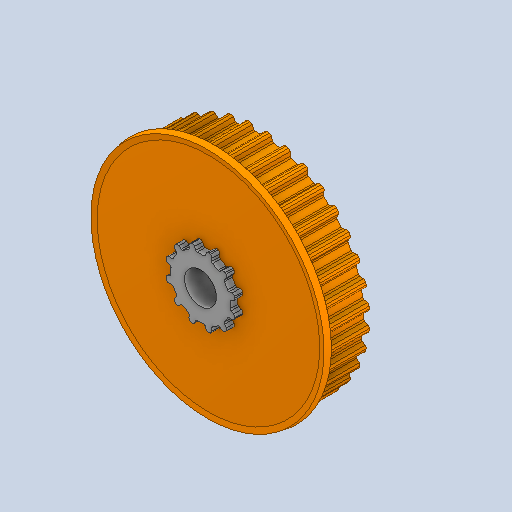
# Autodesk Inventor part: Synchronous Pulley2
Saved by Autodesk Inventor 2022.2 (Build 262287000, 287)
## iProperties
CustomPartVersion: 1
Created: 2022-01-04
Part Number: Synchronous Pulley2
Material: Steel
Document SubType Name: Modeling
Designer: Jochen
Density: 1 g/cm^3
Appearance: Steel
Author: Jochen
Autodesk Inventor part; units mm, degrees
ref_plane "YZ Plane" through (0, 0, 0) normal (1, 0, 0) x (0, 1, 0)
ref_plane "XZ Plane" through (0, 0, 0) normal (0, 1, 0) x (-1, 0, 0)
ref_plane "XY Plane" through (0, 0, 0) normal (0, 0, 1) x (1, 0, 0)
sketch "Pulley Sketch" plane through (0, 0, 0) normal (0, 0, 1) x (1, 0, 0)
  circle A0 centre (0, 0) radius 14.3239 construction
  circle A1 centre (0, 0) radius 14.0239
  circle A2 centre (0, 0) radius 13.2739
  line L0 (-0.8624, 13.9974) -> (-0.525, 13.2739)
  line L1 (-0.525, 13.2739) -> (0.525, 13.2739)
  line L2 (0.525, 13.2739) -> (0.8624, 13.9974)
  line L3 (0, 0) -> (0, 14.0239) construction
  point P0 (0, 13.2739)
  dimension "d0" = 28.6479
  dimension "d1" = 0.3
  dimension "d2" = 0.75
  dimension "d3" = 50
  dimension "d4" = 1.05
  constraints: 8 end point, 3 coincident, 3 point on circle, 2 centre point, 1 horizontal, 1 midpoint, 1 point on line, 1 vertical, 1 vertical alignment, 3 other
  measures "d0" diameter of A0
  measures "d1" radial gap between concentric circles of A0 A1
  measures "d3" angle of L2 L0
  measures "d4" distance of L0.end L1.end
extrude "Base Body" add sketch "Pulley Sketch" along normal mid plane 5.5 contours A2 | A1 L0 L1 L2 | L2 L1 L0 A1
extrude "Tooth" cut sketch "Pulley Sketch" along normal through all both and the other way through all contours L2 L1 L0 A1 picked at (0, 13.7719)
fillet "Tooth Fillet" radius 0.2 2 edges at (0.525, 13.2739, 0) (-0.525, 13.2739, 0)
fillet "Tooth Fillet" radius 0.3 4 edges at (-0.8624, 13.9974, 1.375) (-0.8624, 13.9974, -1.375) (0.8624, 13.9974, 1.375) (0.8624, 13.9974, -1.375)
pattern_circular "Teeth" count 36 over 360 about axis through (0, 0, -10) along (0, 0, 1) of "Tooth", "Tooth Fillet"
feature "Left flange" [suppressed]
pulley flange "Right flange" diameter 28.0479 height 0.8 thickness 0.8 bend angle 10 centre (0, 0, 2.75) toward (0, 0, 1)
sketch "Sketch2" plane through (0, 0, -2.75) normal (0, 0, -1) x (-1, 0, 0)
  circle A0 centre (0, 0) radius 17.5
  circle A1 centre (0, 0) radius 2
  arc A2 (-3.1617, 13.4663) -> (-3.482, 13.5848) centre (-3.4075, 13.2942) ccw projected
  arc A3 (-3.482, 13.5848) -> (-3.7769, 13.5058) centre (0, 0) ccw projected
  arc A4 (-3.7769, 13.5058) -> (-3.995, 13.243) centre (-3.6961, 13.2169) ccw projected
  line L0 (-3.995, 13.243) -> (-4.0355, 12.7799) projected
  arc A5 (-4.1663, 12.6094) -> (-4.0355, 12.7799) centre (-4.2348, 12.7973) ccw projected
  line L1 (-4.1663, 12.6094) -> (-4.9136, 12.3374) projected
  arc A6 (-5.1234, 12.384) -> (-4.9136, 12.3374) centre (-4.982, 12.5254) ccw projected
  line L2 (-5.1234, 12.384) -> (-5.4521, 12.7127) projected
  arc A7 (-5.4521, 12.7127) -> (-5.788, 12.7738) centre (-5.6642, 12.5005) ccw projected
  arc A8 (-5.788, 12.7738) -> (-6.0648, 12.6447) centre (0, 0) ccw projected
  arc A9 (-6.0648, 12.6447) -> (-6.2339, 12.3481) centre (-5.9351, 12.3742) ccw projected
  line L3 (-6.2339, 12.3481) -> (-6.1934, 11.885) projected
  arc A10 (-6.2927, 11.6944) -> (-6.1934, 11.885) centre (-6.3927, 11.8676) ccw projected
  line L4 (-6.2927, 11.6944) -> (-6.9813, 11.2968) projected
  arc A11 (-7.196, 11.3062) -> (-6.9813, 11.2968) centre (-7.0813, 11.47) ccw projected
  line L5 (-7.196, 11.3062) -> (-7.5768, 11.5728) projected
  arc A12 (-7.5768, 11.5728) -> (-7.9183, 11.5746) centre (-7.7489, 11.327) ccw projected
  arc A13 (-7.9183, 11.5746) -> (-8.1684, 11.3995) centre (0, 0) ccw projected
  arc A14 (-8.1684, 11.3995) -> (-8.2834, 11.078) centre (-7.9937, 11.1556) ccw projected
  line L6 (-8.2834, 11.078) -> (-8.1631, 10.629) projected
  arc A15 (-8.2278, 10.424) -> (-8.1631, 10.629) centre (-8.3563, 10.5772) ccw projected
  line L7 (-8.2278, 10.424) -> (-8.8369, 9.9129) projected
  arc A16 (-9.05, 9.8848) -> (-8.8369, 9.9129) centre (-8.9655, 10.0661) ccw projected
  line L8 (-9.05, 9.8848) -> (-9.4713, 10.0813) projected
  arc A17 (-9.4713, 10.0813) -> (-9.8079, 10.0238) centre (-9.5981, 9.8094) ccw projected
  arc A18 (-9.8079, 10.0238) -> (-10.0238, 9.8079) centre (0, 0) ccw projected
  arc A19 (-10.0238, 9.8079) -> (-10.0813, 9.4713) centre (-9.8094, 9.5981) ccw projected
  line L9 (-10.0813, 9.4713) -> (-9.8848, 9.05) projected
  arc A20 (-9.9129, 8.8369) -> (-9.8848, 9.05) centre (-10.0661, 8.9655) ccw projected
  line L10 (-9.9129, 8.8369) -> (-10.424, 8.2278) projected
  arc A21 (-10.629, 8.1631) -> (-10.424, 8.2278) centre (-10.5772, 8.3563) ccw projected
  line L11 (-10.629, 8.1631) -> (-11.078, 8.2834) projected
  arc A22 (-11.078, 8.2834) -> (-11.3995, 8.1684) centre (-11.1556, 7.9937) ccw projected
  arc A23 (-11.3995, 8.1684) -> (-11.5746, 7.9183) centre (0, 0) ccw projected
  arc A24 (-11.5746, 7.9183) -> (-11.5728, 7.5768) centre (-11.327, 7.7489) ccw projected
  line L12 (-11.5728, 7.5768) -> (-11.3062, 7.196) projected
  arc A25 (-11.2968, 6.9813) -> (-11.3062, 7.196) centre (-11.47, 7.0813) ccw projected
  line L13 (-11.2968, 6.9813) -> (-11.6944, 6.2927) projected
  arc A26 (-11.885, 6.1934) -> (-11.6944, 6.2927) centre (-11.8676, 6.3927) ccw projected
  line L14 (-11.885, 6.1934) -> (-12.3481, 6.2339) projected
  arc A27 (-12.3481, 6.2339) -> (-12.6447, 6.0648) centre (-12.3742, 5.9351) ccw projected
  arc A28 (-12.6447, 6.0648) -> (-12.7738, 5.788) centre (0, 0) ccw projected
  arc A29 (-12.7738, 5.788) -> (-12.7127, 5.4521) centre (-12.5005, 5.6642) ccw projected
  line L15 (-12.7127, 5.4521) -> (-12.384, 5.1234) projected
  arc A30 (-12.3374, 4.9136) -> (-12.384, 5.1234) centre (-12.5254, 4.982) ccw projected
  line L16 (-12.3374, 4.9136) -> (-12.6094, 4.1663) projected
  arc A31 (-12.7799, 4.0355) -> (-12.6094, 4.1663) centre (-12.7973, 4.2348) ccw projected
  line L17 (-12.7799, 4.0355) -> (-13.243, 3.995) projected
  arc A32 (-13.243, 3.995) -> (-13.5058, 3.7769) centre (-13.2169, 3.6961) ccw projected
  arc A33 (-13.5058, 3.7769) -> (-13.5848, 3.482) centre (0, 0) ccw projected
  arc A34 (-13.5848, 3.482) -> (-13.4663, 3.1617) centre (-13.2942, 3.4075) ccw projected
  line L18 (-13.4663, 3.1617) -> (-13.0855, 2.8951) projected
  arc A35 (-13.0032, 2.6965) -> (-13.0855, 2.8951) centre (-13.2002, 2.7313) ccw projected
  line L19 (-13.0032, 2.6965) -> (-13.1413, 1.9135) projected
  arc A36 (-13.2865, 1.755) -> (-13.1413, 1.9135) centre (-13.3383, 1.9482) ccw projected
  line L20 (-13.2865, 1.755) -> (-13.7355, 1.6347) projected
  arc A37 (-13.7355, 1.6347) -> (-13.9564, 1.3743) centre (-13.6579, 1.3449) ccw projected
  arc A38 (-13.9564, 1.3743) -> (-13.9831, 1.0701) centre (0, 0) ccw projected
  arc A39 (-13.9831, 1.0701) -> (-13.8107, 0.7753) centre (-13.6839, 1.0472) ccw projected
  line L21 (-13.8107, 0.7753) -> (-13.3894, 0.5788) projected
  arc A40 (-13.2739, 0.3976) -> (-13.3894, 0.5788) centre (-13.4739, 0.3976) ccw projected
  line L22 (-13.2739, 0.3976) -> (-13.2739, -0.3976) projected
  arc A41 (-13.3894, -0.5788) -> (-13.2739, -0.3976) centre (-13.4739, -0.3976) ccw projected
  line L23 (-13.3894, -0.5788) -> (-13.8107, -0.7753) projected
  arc A42 (-13.8107, -0.7753) -> (-13.9831, -1.0701) centre (-13.6839, -1.0472) ccw projected
  arc A43 (-13.9831, -1.0701) -> (-13.9564, -1.3743) centre (0, 0) ccw projected
  arc A44 (-13.9564, -1.3743) -> (-13.7355, -1.6347) centre (-13.6579, -1.3449) ccw projected
  line L24 (-13.7355, -1.6347) -> (-13.2865, -1.755) projected
  arc A45 (-13.1413, -1.9135) -> (-13.2865, -1.755) centre (-13.3383, -1.9482) ccw projected
  line L25 (-13.1413, -1.9135) -> (-13.0032, -2.6965) projected
  arc A46 (-13.0855, -2.8951) -> (-13.0032, -2.6965) centre (-13.2002, -2.7313) ccw projected
  line L26 (-13.0855, -2.8951) -> (-13.4663, -3.1617) projected
  arc A47 (-13.4663, -3.1617) -> (-13.5848, -3.482) centre (-13.2942, -3.4075) ccw projected
  arc A48 (-13.5848, -3.482) -> (-13.5058, -3.7769) centre (0, 0) ccw projected
  arc A49 (-13.5058, -3.7769) -> (-13.243, -3.995) centre (-13.2169, -3.6961) ccw projected
  line L27 (-13.243, -3.995) -> (-12.7799, -4.0355) projected
  arc A50 (-12.6094, -4.1663) -> (-12.7799, -4.0355) centre (-12.7973, -4.2348) ccw projected
  line L28 (-12.6094, -4.1663) -> (-12.3374, -4.9136) projected
  arc A51 (-12.384, -5.1234) -> (-12.3374, -4.9136) centre (-12.5254, -4.982) ccw projected
  line L29 (-12.384, -5.1234) -> (-12.7127, -5.4521) projected
  arc A52 (-12.7127, -5.4521) -> (-12.7738, -5.788) centre (-12.5005, -5.6642) ccw projected
  arc A53 (-12.7738, -5.788) -> (-12.6447, -6.0648) centre (0, 0) ccw projected
  arc A54 (-12.6447, -6.0648) -> (-12.3481, -6.2339) centre (-12.3742, -5.9351) ccw projected
  line L30 (-12.3481, -6.2339) -> (-11.885, -6.1934) projected
  arc A55 (-11.6944, -6.2927) -> (-11.885, -6.1934) centre (-11.8676, -6.3927) ccw projected
  line L31 (-11.6944, -6.2927) -> (-11.2968, -6.9813) projected
  arc A56 (-11.3062, -7.196) -> (-11.2968, -6.9813) centre (-11.47, -7.0813) ccw projected
  line L32 (-11.3062, -7.196) -> (-11.5728, -7.5768) projected
  arc A57 (-11.5728, -7.5768) -> (-11.5746, -7.9183) centre (-11.327, -7.7489) ccw projected
  arc A58 (-11.5746, -7.9183) -> (-11.3995, -8.1684) centre (0, 0) ccw projected
  arc A59 (-11.3995, -8.1684) -> (-11.078, -8.2834) centre (-11.1556, -7.9937) ccw projected
  line L33 (-11.078, -8.2834) -> (-10.629, -8.1631) projected
  arc A60 (-10.424, -8.2278) -> (-10.629, -8.1631) centre (-10.5772, -8.3563) ccw projected
  line L34 (-10.424, -8.2278) -> (-9.9129, -8.8369) projected
  arc A61 (-9.8848, -9.05) -> (-9.9129, -8.8369) centre (-10.0661, -8.9655) ccw projected
  line L35 (-9.8848, -9.05) -> (-10.0813, -9.4713) projected
  arc A62 (-10.0813, -9.4713) -> (-10.0238, -9.8079) centre (-9.8094, -9.5981) ccw projected
  arc A63 (-10.0238, -9.8079) -> (-9.8079, -10.0238) centre (0, 0) ccw projected
  arc A64 (-9.8079, -10.0238) -> (-9.4713, -10.0813) centre (-9.5981, -9.8094) ccw projected
  line L36 (-9.4713, -10.0813) -> (-9.05, -9.8848) projected
  arc A65 (-8.8369, -9.9129) -> (-9.05, -9.8848) centre (-8.9655, -10.0661) ccw projected
  line L37 (-8.8369, -9.9129) -> (-8.2278, -10.424) projected
  arc A66 (-8.1631, -10.629) -> (-8.2278, -10.424) centre (-8.3563, -10.5772) ccw projected
  line L38 (-8.1631, -10.629) -> (-8.2834, -11.078) projected
  arc A67 (-8.2834, -11.078) -> (-8.1684, -11.3995) centre (-7.9937, -11.1556) ccw projected
  arc A68 (-8.1684, -11.3995) -> (-7.9183, -11.5746) centre (0, 0) ccw projected
  arc A69 (-7.9183, -11.5746) -> (-7.5768, -11.5728) centre (-7.7489, -11.327) ccw projected
  line L39 (-7.5768, -11.5728) -> (-7.196, -11.3062) projected
  arc A70 (-6.9813, -11.2968) -> (-7.196, -11.3062) centre (-7.0813, -11.47) ccw projected
  line L40 (-6.9813, -11.2968) -> (-6.2927, -11.6944) projected
  arc A71 (-6.1934, -11.885) -> (-6.2927, -11.6944) centre (-6.3927, -11.8676) ccw projected
  line L41 (-6.1934, -11.885) -> (-6.2339, -12.3481) projected
  arc A72 (-6.2339, -12.3481) -> (-6.0648, -12.6447) centre (-5.9351, -12.3742) ccw projected
  arc A73 (-6.0648, -12.6447) -> (-5.788, -12.7738) centre (0, 0) ccw projected
  arc A74 (-5.788, -12.7738) -> (-5.4521, -12.7127) centre (-5.6642, -12.5005) ccw projected
  line L42 (-5.4521, -12.7127) -> (-5.1234, -12.384) projected
  arc A75 (-4.9136, -12.3374) -> (-5.1234, -12.384) centre (-4.982, -12.5254) ccw projected
  line L43 (-4.9136, -12.3374) -> (-4.1663, -12.6094) projected
  arc A76 (-4.0355, -12.7799) -> (-4.1663, -12.6094) centre (-4.2348, -12.7973) ccw projected
  line L44 (-4.0355, -12.7799) -> (-3.995, -13.243) projected
  arc A77 (-3.995, -13.243) -> (-3.7769, -13.5058) centre (-3.6961, -13.2169) ccw projected
  arc A78 (-3.7769, -13.5058) -> (-3.482, -13.5848) centre (0, 0) ccw projected
  arc A79 (-3.482, -13.5848) -> (-3.1617, -13.4663) centre (-3.4075, -13.2942) ccw projected
  line L45 (-3.1617, -13.4663) -> (-2.8951, -13.0855) projected
  arc A80 (-2.6965, -13.0032) -> (-2.8951, -13.0855) centre (-2.7313, -13.2002) ccw projected
  line L46 (-2.6965, -13.0032) -> (-1.9135, -13.1413) projected
  arc A81 (-1.755, -13.2865) -> (-1.9135, -13.1413) centre (-1.9482, -13.3383) ccw projected
  line L47 (-1.755, -13.2865) -> (-1.6347, -13.7355) projected
  arc A82 (-1.6347, -13.7355) -> (-1.3743, -13.9564) centre (-1.3449, -13.6579) ccw projected
  arc A83 (-1.3743, -13.9564) -> (-1.0701, -13.9831) centre (0, 0) ccw projected
  arc A84 (-1.0701, -13.9831) -> (-0.7753, -13.8107) centre (-1.0472, -13.6839) ccw projected
  line L48 (-0.7753, -13.8107) -> (-0.5788, -13.3894) projected
  arc A85 (-0.3976, -13.2739) -> (-0.5788, -13.3894) centre (-0.3976, -13.4739) ccw projected
  line L49 (-0.3976, -13.2739) -> (0.3976, -13.2739) projected
  arc A86 (0.5788, -13.3894) -> (0.3976, -13.2739) centre (0.3976, -13.4739) ccw projected
  line L50 (0.5788, -13.3894) -> (0.7753, -13.8107) projected
  arc A87 (0.7753, -13.8107) -> (1.0701, -13.9831) centre (1.0472, -13.6839) ccw projected
  arc A88 (1.0701, -13.9831) -> (1.3743, -13.9564) centre (0, 0) ccw projected
  arc A89 (1.3743, -13.9564) -> (1.6347, -13.7355) centre (1.3449, -13.6579) ccw projected
  line L51 (1.6347, -13.7355) -> (1.755, -13.2865) projected
  arc A90 (1.9135, -13.1413) -> (1.755, -13.2865) centre (1.9482, -13.3383) ccw projected
  line L52 (1.9135, -13.1413) -> (2.6965, -13.0032) projected
  arc A91 (2.8951, -13.0855) -> (2.6965, -13.0032) centre (2.7313, -13.2002) ccw projected
  line L53 (2.8951, -13.0855) -> (3.1617, -13.4663) projected
  arc A92 (3.1617, -13.4663) -> (3.482, -13.5848) centre (3.4075, -13.2942) ccw projected
  arc A93 (3.482, -13.5848) -> (3.7769, -13.5058) centre (0, 0) ccw projected
  arc A94 (3.7769, -13.5058) -> (3.995, -13.243) centre (3.6961, -13.2169) ccw projected
  line L54 (3.995, -13.243) -> (4.0355, -12.7799) projected
  arc A95 (4.1663, -12.6094) -> (4.0355, -12.7799) centre (4.2348, -12.7973) ccw projected
  line L55 (4.1663, -12.6094) -> (4.9136, -12.3374) projected
  arc A96 (5.1234, -12.384) -> (4.9136, -12.3374) centre (4.982, -12.5254) ccw projected
  line L56 (5.1234, -12.384) -> (5.4521, -12.7127) projected
  arc A97 (5.4521, -12.7127) -> (5.788, -12.7738) centre (5.6642, -12.5005) ccw projected
  arc A98 (5.788, -12.7738) -> (6.0648, -12.6447) centre (0, 0) ccw projected
  arc A99 (6.0648, -12.6447) -> (6.2339, -12.3481) centre (5.9351, -12.3742) ccw projected
  line L57 (6.2339, -12.3481) -> (6.1934, -11.885) projected
  arc A100 (6.2927, -11.6944) -> (6.1934, -11.885) centre (6.3927, -11.8676) ccw projected
  line L58 (6.2927, -11.6944) -> (6.9813, -11.2968) projected
  arc A101 (7.196, -11.3062) -> (6.9813, -11.2968) centre (7.0813, -11.47) ccw projected
  line L59 (7.196, -11.3062) -> (7.5768, -11.5728) projected
  arc A102 (7.5768, -11.5728) -> (7.9183, -11.5746) centre (7.7489, -11.327) ccw projected
  arc A103 (7.9183, -11.5746) -> (8.1684, -11.3995) centre (0, 0) ccw projected
  arc A104 (8.1684, -11.3995) -> (8.2834, -11.078) centre (7.9937, -11.1556) ccw projected
  line L60 (8.2834, -11.078) -> (8.1631, -10.629) projected
  arc A105 (8.2278, -10.424) -> (8.1631, -10.629) centre (8.3563, -10.5772) ccw projected
  line L61 (8.2278, -10.424) -> (8.8369, -9.9129) projected
  arc A106 (9.05, -9.8848) -> (8.8369, -9.9129) centre (8.9655, -10.0661) ccw projected
  line L62 (9.05, -9.8848) -> (9.4713, -10.0813) projected
  arc A107 (9.4713, -10.0813) -> (9.8079, -10.0238) centre (9.5981, -9.8094) ccw projected
  arc A108 (9.8079, -10.0238) -> (10.0238, -9.8079) centre (0, 0) ccw projected
  arc A109 (10.0238, -9.8079) -> (10.0813, -9.4713) centre (9.8094, -9.5981) ccw projected
  line L63 (10.0813, -9.4713) -> (9.8848, -9.05) projected
  arc A110 (9.9129, -8.8369) -> (9.8848, -9.05) centre (10.0661, -8.9655) ccw projected
  line L64 (9.9129, -8.8369) -> (10.424, -8.2278) projected
  arc A111 (10.629, -8.1631) -> (10.424, -8.2278) centre (10.5772, -8.3563) ccw projected
  line L65 (10.629, -8.1631) -> (11.078, -8.2834) projected
  arc A112 (11.078, -8.2834) -> (11.3995, -8.1684) centre (11.1556, -7.9937) ccw projected
  arc A113 (11.3995, -8.1684) -> (11.5746, -7.9183) centre (0, 0) ccw projected
  arc A114 (11.5746, -7.9183) -> (11.5728, -7.5768) centre (11.327, -7.7489) ccw projected
  line L66 (11.5728, -7.5768) -> (11.3062, -7.196) projected
  arc A115 (11.2968, -6.9813) -> (11.3062, -7.196) centre (11.47, -7.0813) ccw projected
  line L67 (11.2968, -6.9813) -> (11.6944, -6.2927) projected
  arc A116 (11.885, -6.1934) -> (11.6944, -6.2927) centre (11.8676, -6.3927) ccw projected
  line L68 (11.885, -6.1934) -> (12.3481, -6.2339) projected
  arc A117 (12.3481, -6.2339) -> (12.6447, -6.0648) centre (12.3742, -5.9351) ccw projected
  arc A118 (12.6447, -6.0648) -> (12.7738, -5.788) centre (0, 0) ccw projected
  arc A119 (12.7738, -5.788) -> (12.7127, -5.4521) centre (12.5005, -5.6642) ccw projected
  line L69 (12.7127, -5.4521) -> (12.384, -5.1234) projected
  arc A120 (12.3374, -4.9136) -> (12.384, -5.1234) centre (12.5254, -4.982) ccw projected
  line L70 (12.3374, -4.9136) -> (12.6094, -4.1663) projected
  arc A121 (12.7799, -4.0355) -> (12.6094, -4.1663) centre (12.7973, -4.2348) ccw projected
  line L71 (12.7799, -4.0355) -> (13.243, -3.995) projected
  arc A122 (13.243, -3.995) -> (13.5058, -3.7769) centre (13.2169, -3.6961) ccw projected
  arc A123 (13.5058, -3.7769) -> (13.5848, -3.482) centre (0, 0) ccw projected
  arc A124 (13.5848, -3.482) -> (13.4663, -3.1617) centre (13.2942, -3.4075) ccw projected
  line L72 (13.4663, -3.1617) -> (13.0855, -2.8951) projected
  arc A125 (13.0032, -2.6965) -> (13.0855, -2.8951) centre (13.2002, -2.7313) ccw projected
  line L73 (13.0032, -2.6965) -> (13.1413, -1.9135) projected
  arc A126 (13.2865, -1.755) -> (13.1413, -1.9135) centre (13.3383, -1.9482) ccw projected
  line L74 (13.2865, -1.755) -> (13.7355, -1.6347) projected
  arc A127 (13.7355, -1.6347) -> (13.9564, -1.3743) centre (13.6579, -1.3449) ccw projected
  arc A128 (13.9564, -1.3743) -> (13.9831, -1.0701) centre (0, 0) ccw projected
  arc A129 (13.9831, -1.0701) -> (13.8107, -0.7753) centre (13.6839, -1.0472) ccw projected
  line L75 (13.8107, -0.7753) -> (13.3894, -0.5788) projected
  arc A130 (13.2739, -0.3976) -> (13.3894, -0.5788) centre (13.4739, -0.3976) ccw projected
  line L76 (13.2739, -0.3976) -> (13.2739, 0.3976) projected
  arc A131 (13.3894, 0.5788) -> (13.2739, 0.3976) centre (13.4739, 0.3976) ccw projected
  line L77 (13.3894, 0.5788) -> (13.8107, 0.7753) projected
  arc A132 (13.8107, 0.7753) -> (13.9831, 1.0701) centre (13.6839, 1.0472) ccw projected
  arc A133 (13.9831, 1.0701) -> (13.9564, 1.3743) centre (0, 0) ccw projected
  arc A134 (13.9564, 1.3743) -> (13.7355, 1.6347) centre (13.6579, 1.3449) ccw projected
  line L78 (13.7355, 1.6347) -> (13.2865, 1.755) projected
  arc A135 (13.1413, 1.9135) -> (13.2865, 1.755) centre (13.3383, 1.9482) ccw projected
  line L79 (13.1413, 1.9135) -> (13.0032, 2.6965) projected
  arc A136 (13.0855, 2.8951) -> (13.0032, 2.6965) centre (13.2002, 2.7313) ccw projected
  line L80 (13.0855, 2.8951) -> (13.4663, 3.1617) projected
  arc A137 (13.4663, 3.1617) -> (13.5848, 3.482) centre (13.2942, 3.4075) ccw projected
  arc A138 (13.5848, 3.482) -> (13.5058, 3.7769) centre (0, 0) ccw projected
  arc A139 (13.5058, 3.7769) -> (13.243, 3.995) centre (13.2169, 3.6961) ccw projected
  line L81 (13.243, 3.995) -> (12.7799, 4.0355) projected
  arc A140 (12.6094, 4.1663) -> (12.7799, 4.0355) centre (12.7973, 4.2348) ccw projected
  line L82 (12.6094, 4.1663) -> (12.3374, 4.9136) projected
  arc A141 (12.384, 5.1234) -> (12.3374, 4.9136) centre (12.5254, 4.982) ccw projected
  line L83 (12.384, 5.1234) -> (12.7127, 5.4521) projected
  arc A142 (12.7127, 5.4521) -> (12.7738, 5.788) centre (12.5005, 5.6642) ccw projected
  arc A143 (12.7738, 5.788) -> (12.6447, 6.0648) centre (0, 0) ccw projected
  arc A144 (12.6447, 6.0648) -> (12.3481, 6.2339) centre (12.3742, 5.9351) ccw projected
  line L84 (12.3481, 6.2339) -> (11.885, 6.1934) projected
  arc A145 (11.6944, 6.2927) -> (11.885, 6.1934) centre (11.8676, 6.3927) ccw projected
  line L85 (11.6944, 6.2927) -> (11.2968, 6.9813) projected
  arc A146 (11.3062, 7.196) -> (11.2968, 6.9813) centre (11.47, 7.0813) ccw projected
  line L86 (11.3062, 7.196) -> (11.5728, 7.5768) projected
  arc A147 (11.5728, 7.5768) -> (11.5746, 7.9183) centre (11.327, 7.7489) ccw projected
  arc A148 (11.5746, 7.9183) -> (11.3995, 8.1684) centre (0, 0) ccw projected
  arc A149 (11.3995, 8.1684) -> (11.078, 8.2834) centre (11.1556, 7.9937) ccw projected
  line L87 (11.078, 8.2834) -> (10.629, 8.1631) projected
  arc A150 (10.424, 8.2278) -> (10.629, 8.1631) centre (10.5772, 8.3563) ccw projected
  line L88 (10.424, 8.2278) -> (9.9129, 8.8369) projected
  arc A151 (9.8848, 9.05) -> (9.9129, 8.8369) centre (10.0661, 8.9655) ccw projected
  line L89 (9.8848, 9.05) -> (10.0813, 9.4713) projected
  arc A152 (10.0813, 9.4713) -> (10.0238, 9.8079) centre (9.8094, 9.5981) ccw projected
  arc A153 (10.0238, 9.8079) -> (9.8079, 10.0238) centre (0, 0) ccw projected
  arc A154 (9.8079, 10.0238) -> (9.4713, 10.0813) centre (9.5981, 9.8094) ccw projected
  line L90 (9.4713, 10.0813) -> (9.05, 9.8848) projected
  arc A155 (8.8369, 9.9129) -> (9.05, 9.8848) centre (8.9655, 10.0661) ccw projected
  line L91 (8.8369, 9.9129) -> (8.2278, 10.424) projected
  arc A156 (8.1631, 10.629) -> (8.2278, 10.424) centre (8.3563, 10.5772) ccw projected
  line L92 (8.1631, 10.629) -> (8.2834, 11.078) projected
  arc A157 (8.2834, 11.078) -> (8.1684, 11.3995) centre (7.9937, 11.1556) ccw projected
  arc A158 (8.1684, 11.3995) -> (7.9183, 11.5746) centre (0, 0) ccw projected
  arc A159 (7.9183, 11.5746) -> (7.5768, 11.5728) centre (7.7489, 11.327) ccw projected
  line L93 (7.5768, 11.5728) -> (7.196, 11.3062) projected
  arc A160 (6.9813, 11.2968) -> (7.196, 11.3062) centre (7.0813, 11.47) ccw projected
  line L94 (6.9813, 11.2968) -> (6.2927, 11.6944) projected
  arc A161 (6.1934, 11.885) -> (6.2927, 11.6944) centre (6.3927, 11.8676) ccw projected
  line L95 (6.1934, 11.885) -> (6.2339, 12.3481) projected
  arc A162 (6.2339, 12.3481) -> (6.0648, 12.6447) centre (5.9351, 12.3742) ccw projected
  arc A163 (6.0648, 12.6447) -> (5.788, 12.7738) centre (0, 0) ccw projected
  arc A164 (5.788, 12.7738) -> (5.4521, 12.7127) centre (5.6642, 12.5005) ccw projected
  line L96 (5.4521, 12.7127) -> (5.1234, 12.384) projected
  arc A165 (4.9136, 12.3374) -> (5.1234, 12.384) centre (4.982, 12.5254) ccw projected
  line L97 (4.9136, 12.3374) -> (4.1663, 12.6094) projected
  arc A166 (4.0355, 12.7799) -> (4.1663, 12.6094) centre (4.2348, 12.7973) ccw projected
  line L98 (4.0355, 12.7799) -> (3.995, 13.243) projected
  arc A167 (3.995, 13.243) -> (3.7769, 13.5058) centre (3.6961, 13.2169) ccw projected
  arc A168 (3.7769, 13.5058) -> (3.482, 13.5848) centre (0, 0) ccw projected
  arc A169 (3.482, 13.5848) -> (3.1617, 13.4663) centre (3.4075, 13.2942) ccw projected
  line L99 (3.1617, 13.4663) -> (2.8951, 13.0855) projected
  arc A170 (2.6965, 13.0032) -> (2.8951, 13.0855) centre (2.7313, 13.2002) ccw projected
  line L100 (2.6965, 13.0032) -> (1.9135, 13.1413) projected
  arc A171 (1.755, 13.2865) -> (1.9135, 13.1413) centre (1.9482, 13.3383) ccw projected
  line L101 (1.755, 13.2865) -> (1.6347, 13.7355) projected
  arc A172 (1.6347, 13.7355) -> (1.3743, 13.9564) centre (1.3449, 13.6579) ccw projected
  arc A173 (1.3743, 13.9564) -> (1.0701, 13.9831) centre (0, 0) ccw projected
  arc A174 (1.0701, 13.9831) -> (0.7753, 13.8107) centre (1.0472, 13.6839) ccw projected
  line L102 (0.7753, 13.8107) -> (0.5788, 13.3894) projected
  arc A175 (0.3976, 13.2739) -> (0.5788, 13.3894) centre (0.3976, 13.4739) ccw projected
  line L103 (0.3976, 13.2739) -> (-0.3976, 13.2739) projected
  arc A176 (-0.5788, 13.3894) -> (-0.3976, 13.2739) centre (-0.3976, 13.4739) ccw projected
  line L104 (-0.5788, 13.3894) -> (-0.7753, 13.8107) projected
  arc A177 (-0.7753, 13.8107) -> (-1.0701, 13.9831) centre (-1.0472, 13.6839) ccw projected
  arc A178 (-1.0701, 13.9831) -> (-1.3743, 13.9564) centre (0, 0) ccw projected
  arc A179 (-1.3743, 13.9564) -> (-1.6347, 13.7355) centre (-1.3449, 13.6579) ccw projected
  line L105 (-1.6347, 13.7355) -> (-1.755, 13.2865) projected
  arc A180 (-1.9135, 13.1413) -> (-1.755, 13.2865) centre (-1.9482, 13.3383) ccw projected
  line L106 (-1.9135, 13.1413) -> (-2.6965, 13.0032) projected
  arc A181 (-2.8951, 13.0855) -> (-2.6965, 13.0032) centre (-2.7313, 13.2002) ccw projected
  line L107 (-2.8951, 13.0855) -> (-3.1617, 13.4663) projected
  dimension "d17" = 35
  dimension "d24" = 4
  constraints: 2 centre point, 2 coincident
  measures "d17" diameter of A0
  measures "d24" diameter of A1
sketch "Sketch4" plane through (0, 0, -2.75) normal (0, 0, -1) x (-1, 0, 0)
  arc A0 (0.3976, 3.7246) -> (0.5788, 3.8401) centre (0.3976, 3.9246) ccw
  line L0 (0.5788, 3.8401) -> (0.7363, 4.1779)
  arc A1 (1.0807, 4.3422) -> (0.7363, 4.1779) centre (1.0082, 4.0511) ccw
  arc A2 (1.2352, 4.3008) -> (1.0807, 4.3422) centre (0, 0) ccw
  arc A3 (1.4512, 3.9863) -> (1.2352, 4.3008) centre (1.1524, 4.0124) ccw
  line L1 (1.4512, 3.9863) -> (1.4188, 3.6151)
  arc A4 (1.4188, 3.6151) -> (1.518, 3.4244) centre (1.618, 3.5976) ccw
  line L2 (1.518, 3.4244) -> (2.2066, 3.0268)
  arc A5 (2.2066, 3.0268) -> (2.4214, 3.0362) centre (2.3066, 3.2001) ccw
  line L3 (2.4214, 3.0362) -> (2.7266, 3.25)
  arc A6 (3.107, 3.2201) -> (2.7266, 3.25) centre (2.8987, 3.0042) ccw
  arc A7 (3.2201, 3.107) -> (3.107, 3.2201) centre (0, 0) ccw
  arc A8 (3.25, 2.7266) -> (3.2201, 3.107) centre (3.0042, 2.8987) ccw
  line L4 (3.25, 2.7266) -> (3.0362, 2.4214)
  arc A9 (3.0362, 2.4214) -> (3.0268, 2.2066) centre (3.2001, 2.3066) ccw
  line L5 (3.0268, 2.2066) -> (3.4244, 1.518)
  arc A10 (3.4244, 1.518) -> (3.6151, 1.4188) centre (3.5976, 1.618) ccw
  line L6 (3.6151, 1.4188) -> (3.9863, 1.4512)
  arc A11 (4.3008, 1.2352) -> (3.9863, 1.4512) centre (4.0124, 1.1524) ccw
  arc A12 (4.3422, 1.0807) -> (4.3008, 1.2352) centre (0, 0) ccw
  arc A13 (4.1779, 0.7363) -> (4.3422, 1.0807) centre (4.0511, 1.0082) ccw
  line L7 (4.1779, 0.7363) -> (3.8401, 0.5788)
  arc A14 (3.8401, 0.5788) -> (3.7246, 0.3976) centre (3.9246, 0.3976) ccw
  line L8 (3.7246, 0.3976) -> (3.7246, -0.3976)
  arc A15 (3.7246, -0.3976) -> (3.8401, -0.5788) centre (3.9246, -0.3976) ccw
  line L9 (3.8401, -0.5788) -> (4.1779, -0.7363)
  arc A16 (4.3422, -1.0807) -> (4.1779, -0.7363) centre (4.0511, -1.0082) ccw
  arc A17 (4.3008, -1.2352) -> (4.3422, -1.0807) centre (0, 0) ccw
  arc A18 (3.9863, -1.4512) -> (4.3008, -1.2352) centre (4.0124, -1.1524) ccw
  line L10 (3.9863, -1.4512) -> (3.6151, -1.4188)
  arc A19 (3.6151, -1.4188) -> (3.4244, -1.518) centre (3.5976, -1.618) ccw
  line L11 (3.4244, -1.518) -> (3.0268, -2.2066)
  arc A20 (3.0268, -2.2066) -> (3.0362, -2.4214) centre (3.2001, -2.3066) ccw
  line L12 (3.0362, -2.4214) -> (3.25, -2.7266)
  arc A21 (3.2201, -3.107) -> (3.25, -2.7266) centre (3.0042, -2.8987) ccw
  arc A22 (3.107, -3.2201) -> (3.2201, -3.107) centre (0, 0) ccw
  arc A23 (2.7266, -3.25) -> (3.107, -3.2201) centre (2.8987, -3.0042) ccw
  line L13 (2.7266, -3.25) -> (2.4214, -3.0362)
  arc A24 (2.4214, -3.0362) -> (2.2066, -3.0268) centre (2.3066, -3.2001) ccw
  line L14 (2.2066, -3.0268) -> (1.518, -3.4244)
  arc A25 (1.518, -3.4244) -> (1.4188, -3.6151) centre (1.618, -3.5976) ccw
  line L15 (1.4188, -3.6151) -> (1.4512, -3.9863)
  arc A26 (1.2352, -4.3008) -> (1.4512, -3.9863) centre (1.1524, -4.0124) ccw
  arc A27 (1.0807, -4.3422) -> (1.2352, -4.3008) centre (0, 0) ccw
  arc A28 (0.7363, -4.1779) -> (1.0807, -4.3422) centre (1.0082, -4.0511) ccw
  line L16 (0.7363, -4.1779) -> (0.5788, -3.8401)
  arc A29 (0.5788, -3.8401) -> (0.3976, -3.7246) centre (0.3976, -3.9246) ccw
  line L17 (0.3976, -3.7246) -> (-0.3976, -3.7246)
  arc A30 (-0.3976, -3.7246) -> (-0.5788, -3.8401) centre (-0.3976, -3.9246) ccw
  line L18 (-0.5788, -3.8401) -> (-0.7363, -4.1779)
  arc A31 (-1.0807, -4.3422) -> (-0.7363, -4.1779) centre (-1.0082, -4.0511) ccw
  arc A32 (-1.2352, -4.3008) -> (-1.0807, -4.3422) centre (0, 0) ccw
  arc A33 (-1.4512, -3.9863) -> (-1.2352, -4.3008) centre (-1.1524, -4.0124) ccw
  line L19 (-1.4512, -3.9863) -> (-1.4188, -3.6151)
  arc A34 (-1.4188, -3.6151) -> (-1.518, -3.4244) centre (-1.618, -3.5976) ccw
  line L20 (-1.518, -3.4244) -> (-2.2066, -3.0268)
  arc A35 (-2.2066, -3.0268) -> (-2.4214, -3.0362) centre (-2.3066, -3.2001) ccw
  line L21 (-2.4214, -3.0362) -> (-2.7266, -3.25)
  arc A36 (-3.107, -3.2201) -> (-2.7266, -3.25) centre (-2.8987, -3.0042) ccw
  arc A37 (-3.2201, -3.107) -> (-3.107, -3.2201) centre (0, 0) ccw
  arc A38 (-3.25, -2.7266) -> (-3.2201, -3.107) centre (-3.0042, -2.8987) ccw
  line L22 (-3.25, -2.7266) -> (-3.0362, -2.4214)
  arc A39 (-3.0362, -2.4214) -> (-3.0268, -2.2066) centre (-3.2001, -2.3066) ccw
  line L23 (-3.0268, -2.2066) -> (-3.4244, -1.518)
  arc A40 (-3.4244, -1.518) -> (-3.6151, -1.4188) centre (-3.5976, -1.618) ccw
  line L24 (-3.6151, -1.4188) -> (-3.9863, -1.4512)
  arc A41 (-4.3008, -1.2352) -> (-3.9863, -1.4512) centre (-4.0124, -1.1524) ccw
  arc A42 (-4.3422, -1.0807) -> (-4.3008, -1.2352) centre (0, 0) ccw
  arc A43 (-4.1779, -0.7363) -> (-4.3422, -1.0807) centre (-4.0511, -1.0082) ccw
  line L25 (-4.1779, -0.7363) -> (-3.8401, -0.5788)
  arc A44 (-3.8401, -0.5788) -> (-3.7246, -0.3976) centre (-3.9246, -0.3976) ccw
  line L26 (-3.7246, -0.3976) -> (-3.7246, 0.3976)
  arc A45 (-3.7246, 0.3976) -> (-3.8401, 0.5788) centre (-3.9246, 0.3976) ccw
  line L27 (-3.8401, 0.5788) -> (-4.1779, 0.7363)
  arc A46 (-4.3422, 1.0807) -> (-4.1779, 0.7363) centre (-4.0511, 1.0082) ccw
  arc A47 (-4.3008, 1.2352) -> (-4.3422, 1.0807) centre (0, 0) ccw
  arc A48 (-3.9863, 1.4512) -> (-4.3008, 1.2352) centre (-4.0124, 1.1524) ccw
  line L28 (-3.9863, 1.4512) -> (-3.6151, 1.4188)
  arc A49 (-3.6151, 1.4188) -> (-3.4244, 1.518) centre (-3.5976, 1.618) ccw
  line L29 (-3.4244, 1.518) -> (-3.0268, 2.2066)
  arc A50 (-3.0268, 2.2066) -> (-3.0362, 2.4214) centre (-3.2001, 2.3066) ccw
  line L30 (-3.0362, 2.4214) -> (-3.25, 2.7266)
  arc A51 (-3.2201, 3.107) -> (-3.25, 2.7266) centre (-3.0042, 2.8987) ccw
  arc A52 (-3.107, 3.2201) -> (-3.2201, 3.107) centre (0, 0) ccw
  arc A53 (-2.7266, 3.25) -> (-3.107, 3.2201) centre (-2.8987, 3.0042) ccw
  line L31 (-2.7266, 3.25) -> (-2.4214, 3.0362)
  arc A54 (-2.4214, 3.0362) -> (-2.2066, 3.0268) centre (-2.3066, 3.2001) ccw
  line L32 (-2.2066, 3.0268) -> (-1.518, 3.4244)
  arc A55 (-1.518, 3.4244) -> (-1.4188, 3.6151) centre (-1.618, 3.5976) ccw
  line L33 (-1.4188, 3.6151) -> (-1.4512, 3.9863)
  arc A56 (-1.2352, 4.3008) -> (-1.4512, 3.9863) centre (-1.1524, 4.0124) ccw
  arc A57 (-1.0807, 4.3422) -> (-1.2352, 4.3008) centre (0, 0) ccw
  arc A58 (-0.7363, 4.1779) -> (-1.0807, 4.3422) centre (-1.0082, 4.0511) ccw
  line L34 (-0.7363, 4.1779) -> (-0.5788, 3.8401)
  arc A59 (-0.5788, 3.8401) -> (-0.3976, 3.7246) centre (-0.3976, 3.9246) ccw
  line L35 (-0.3976, 3.7246) -> (0.3976, 3.7246)
  circle A60 centre (0, 0) radius 5.3798
  constraints: 120 point on circle, 72 end point, 61 centre point, 1 coincident
extrude "Extrusion7" add sketch "Sketch4" along normal blind 1
chamfer "Chamfer1" distance 1.5 distance2 0.5 1 edges at (5.3798, 0, -3.75) measured on face at (4.8798, 0, -3.75)
extrude "Extrusion4" cut sketch "Sketch4" against normal through all contours A0 L0 A1 A2 A3 L1 A4 L2 A5 L3 A6 A7 A8 L4 A9 L5 A10 L6 A11 A12 A13 L7 A14 L8 A15 L9 A16 A17 A18 L10 A19 L11 A20 L12 A21 A22 A23 L13 A24 L14 A25 L15 A26 A27 A28 L16 A29 L17 A30 L18 A31 A32 A33 L19 A34 L20 A35 L21 A36 A37 A38 L22 A39 L23 A40 L24 A41 A42 A43 L25 A44 L26 A45 L27 A46 A47 A48 L28 A49 L29 A50 L30 A51 A52 A53 L31 A54 L32 A55 L33 A56 A57 A58 L34 A59 L35
extrude "Extrusion5" add sketch "Sketch4" along normal blind 13 and the other way blind 1 from surface at -6.3 separate body contours A0 L0 A1 A2 A3 L1 A4 L2 A5 L3 A6 A7 A8 L4 A9 L5 A10 L6 A11 A12 A13 L7 A14 L8 A15 L9 A16 A17 A18 L10 A19 L11 A20 L12 A21 A22 A23 L13 A24 L14 A25 L15 A26 A27 A28 L16 A29 L17 A30 L18 A31 A32 A33 L19 A34 L20 A35 L21 A36 A37 A38 L22 A39 L23 A40 L24 A41 A42 A43 L25 A44 L26 A45 L27 A46 A47 A48 L28 A49 L29 A50 L30 A51 A52 A53 L31 A54 L32 A55 L33 A56 A57 A58 L34 A59 L35
extrude "Extrusion6" cut sketch "Sketch2" along normal through all both and the other way through all contours A1 bodies 2 1
equation "\"d1\" = da_a"
equation "\"d2\" = da_hg"
equation "\"d3\" = 2 * da_fi"
equation "\"d4\" = da_bw"
equation "\"d5\" = da_bf"
equation "\"d7\" = da_bf"
equation "\"d9\" = da_rb"
equation "\"d10\" = da_rt"
equation "\"da_pb\" = 2.5"
equation "\"da_fi\" = 25deg"
equation "\"da_hg\" = 0.75"
equation "\"da_bw\" = 1.05"
equation "\"da_rb\" = 0.2"
equation "\"da_rt\" = 0.3"
equation "\"da_a\" = 0.3"
equation "\"da_bf\" = 5.5"
equation "\"da_wf\" = 0.8"
equation "\"da_hf\" = 0.8"
body "Solid1"
body "Solid2"
